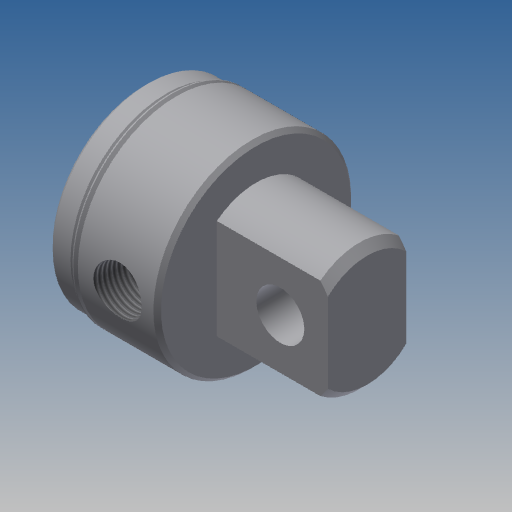
# Autodesk Inventor part: 17P0000_rear_head
Saved by Autodesk Inventor 2020 (Build 240168000, 168)
## iProperties
Created: 2020-02-18
Part Number: 17P0000_rear_head
Material: Generic
Catalog Web Link: www.cadenas.de
Description: Rear Head-Original Line - Standard Air Cylinders
Vendor: BIMBA
Document SubType Name: Modeling
Designer: psadmin
Manufacturer: BIMBA
Mass: 27.57 g
Surface Area: 88.2977 cm^2
Volume: 27.57 cm^3
Density: 1 g/cm^3
Appearance: PSOLRGB-211-211-211
Category: PARTsolutions
Company: BIMBA
PSOL_IDENT_0: {$CADENAS_DATA\23d-libs\bimba\bimba_brand\bimba_imperial\bimba_full_line\original_line_cylinders\sta
PSOL_IDENT_1: ndard_air_cylinders\rear_head.prj},239 {VTYP=3D},{NB=17P0000_rear_head},{LINA=17P0000_rear_head},{NN=
PSOL_IDENT_2: Rear Head},{DATE=10.02.2020 11:56:01},{GEOMDATE=15.10.2019 12:00:43},{VERSION=},{LINEID=80},{WBVAR=M
PSOL_IDENT_3: NT,ACTING,DER,Q,T1,T2,T3,T4,TRIM,Y,K,MB,CUSH,FBON},{WBNUMERIC=TRIM,MB,CUSH}  {NB=17P0000_rear_head},
PSOL_IDENT_4: {LINA=17P0000_rear_head},{KT=DUMMY},{PN=17P0000},{BORE=1.50000},{BOREPN=17},{MNT=P},{MNTALG='' , 'Fr
PSOL_IDENT_5: ont Nose' , 'P' , 'Rear Pivot' , 'S' , 'Built-in Valve S' , 'DX' , 'Double End' , 'A' , 'Adjustable
PSOL_IDENT_6: Stroke' , 'M' , 'Manual Valve' , 'BR' , 'Rear Block' , 'BRT' , 'Rear Trunnion'},{ACTING=},{ACTINGALG=
PSOL_IDENT_7: '' , 'Single Acting' },{DER=},{DERALG= '' , 'Standard' },{Q=},{T1=},{T2=},{T3=},{T4=},{TRIM=0},{Y=}
PSOL_IDENT_8: ,{K=},{KALG= '', 'without K', 'K', 'with K' },{MB=0},{A1=1.7500},{A1N=0.6880},{A1P=1.7500},{A1B=1.37
PSOL_IDENT_9: 50},{A1S=1.5000},{A2=0.25},{A2N=0.2500},{A3=0.0400},{D1=1.5565},{D1N=1.5565},{D1P=1.5565},{D1B=1.580
PSOL_IDENT_10: 0},{D2=1.5115},{C1=0.0300},{C2=0.0300},{NDM=0.4050},{TAB=NPT},{NDMDP=0.2730},{D3=0.3440},{A4=0.2500}
PSOL_IDENT_11: ,{A5=0.8700},{D4=0.9730},{A6=0.2500},{A7=0.6250},{A8=0.0000},{D5=0.0000},{D6=0.5320},{A9=0.7320},{ND
PSOL_IDENT_12: M2=0.0000},{TAB2=-},{C11=0.0300},{C22=0.0000},{C33=0.0000},{C44=0.0300},{A10=0.6170},{A11=0.0000},{N
PSOL_IDENT_13: DM3=0.4050},{NDM3N=0.4050},{NDM3B=0.5400},{TAB3=NPT},{TAB3N=NPT},{TAB3B=NPT},{A12=0.562},{A12N=0.562
PSOL_IDENT_14: 0},{A12B=0.7500},{A13=1.3750},{D7=0.3775},{D8=1.0000},{A14=0.0000},{A15=0.0000},{D9=0.0000},{R1=0.00
PSOL_IDENT_15: 00},{X1=0.9690},{X2=0.2500},{CX=0.0600},{CC=0.0000},{CON=1},{S1=1.7500},{DB=0.4380},{X1B=0.9730},{X2
PSOL_IDENT_16: B=0.2500},{A8B=0.1250},{A9B=1.0620},{MODEL=1},{NDM4=0.2500},{TAB4=UNC},{NDM4DP=0.5000},{BC=1.7500},{
PSOL_IDENT_17: B1=0.8750},{B2=0.3800},{B3=0.5000},{ON=0},{ON2=1},{G1=0.0000},{G2=0.0000},{G3=0.0000},{G4=0.0000},{G
PSOL_IDENT_18: D=0.0000},{G5=0.0000},{G6=0.0000},{RON=0},{H1=1.6160},{H2=1.5800},{H3=0.1250},{H4=0.1250},{H5=1.5300
PSOL_IDENT_19: },{H6=0.8120},{F=0.6240},{PNUT=0.0000},{CUSH=0},{CC11=0.397},{CC111=0.3965},{CC22=0.5625},{CC33=0.30
PSOL_IDENT_20: 50},{CC44=0.6250},{CC55=0.8750},{CD1=0.2650},{CD2=0.1980},{CD3=0.1345},{CNDM3=0.2500},{CTAB3=UNS},{O
PSOL_IDENT_21: LEN=1.3750},{OD=0.5025},{STDIS=0.3184},{STDIS1=0.3184},{BUSHCON=D-624},{BUSHL=0.7500},{FBON=0},{LCD=
PSOL_IDENT_22: 0.0000}
NN: Rear Head
NT: Original Line - Standard Air Cylinders
NB: 17P0000_rear_head
NBSYN: $PN._rear_head
LINA: 17P0000_rear_head
PN: 17P0000
BORE: 1.5
BOREPN: 17
MNT: Rear Pivot
MNTALG: '' , 'Front Nose' , 'P' , 'Rear Pivot' , 'S' , 'Built-in Valve S' , 'DX' , 'Double End' , 'A' , 'Adjustable Stroke' , 'M' , 'Manual Valve' , 'BR' , 'Rear Block' , 'BRT' , 'Rear Trunnion'
ACTING: Single Acting
DER: Standard
Q: Without Side Ported Rear Head
T1: without T1
T2: without T2
T3: without T3
T4: without T4
TRIM: 0
Y: without Pivot Bushing
K: without K
MB: 0
A1N: 0.688
A1P: 1.75
A1B: 1.375
A1S: 1.5
A2N: 0.25
A3: 0.04
D1N: 1.5565
D1P: 1.5565
D1B: 1.58
D2: 1.5115
C1: 0.03
C2: 0.03
TAB: NPT
NDMDP: 0.273
D3: 0.344
A4: 0.25
A5: 0.87
D4: 0.973
A6: 0.25
A7: 0.625
A8: 0
D5: 0
D6: 0.532
A9: 0.732
NDM2: 0
TAB2: -
C11: 0.03
C22: 0
C33: 0
C44: 0.03
A10: 0.617
A11: 0
NDM3N: 0.405
NDM3B: 0.54
TAB3N: NPT
TAB3B: NPT
A12N: 0.562
A12B: 0.75
A13: 1.375
D7: 0.3775
D8: 1
A14: 0
A15: 0
D9: 0
R1: 0
X1: 0.969
X2: 0.25
CX: 0.06
CC: 0
S1: 1.75
DB: 0.438
X1B: 0.973
X2B: 0.25
A8B: 0.125
A9B: 1.062
NDM4: 0.25
TAB4: UNC
NDM4DP: 0.5
BC: 1.75
B1: 0.875
B2: 0.38
B3: 0.5
G1: 0
G2: 0
G3: 0
G4: 0
GD: 0
G5: 0
G6: 0
H2: 1.58
H3: 0.125
F: 0.624
CUSH: 0
CC111: 0.3965
CC22: 0.5625
CC33: 0.305
CC44: 0.625
CC55: 0.875
CD1: 0.265
CD2: 0.198
CD3: 0.1345
CNDM3: 0.25
CTAB3: UNS
OD: 0.5025
STDIS1: 0.3184
BUSHCON: D-624
BUSHL: 0.75
FBON: 0
LCD: 0
SUPPLIER: BIMBA
ARTICLENO: 17P0000_rear_head
BOMINFO: 17P0000_rear_head
CREATOR: CADENAS GmbH
Title: 17P0000_rear_head
Author: Cadenas PARTsolutions
Comments: Original Line - Standard Air Cylinders
Autodesk Inventor part; units mm, degrees
sketch "Sketch_18" plane through (0, 0, 0) normal (0, 0, 1) x (1, 0, 0)
  line L0 (22.225, 0) -> (0, 0)
  line L1 (0, 0) -> (0, 18.434)
  line L2 (0, 18.434) -> (0.762, 19.196)
  line L3 (0.762, 19.196) -> (4.318, 19.196)
  line L4 (4.318, 19.196) -> (5.334, 18.1801)
  line L5 (5.334, 18.1801) -> (6.35, 18.1801)
  line L6 (6.35, 18.1801) -> (6.35, 19.7675)
  line L7 (6.35, 19.7675) -> (21.463, 19.7675)
  line L8 (21.463, 19.7675) -> (22.225, 19.0055)
  line L9 (22.225, 19.0055) -> (22.225, 0)
  line L10 (22.225, 0) -> (0, 0)
  constraints: 22 end point
revolve "Revolution1" add sketch "Sketch_18" angle 360 about axis through (22.225, 0, 0) along (1, 0, 0)
sketch "Sketch_21" plane through (0, 0, 0) normal (0, 0, 1) x (1, 0, 0)
  line L0 (44.45, 0) -> (22.225, 0)
  line L1 (22.225, 0) -> (22.225, 12.7)
  line L2 (22.225, 12.7) -> (42.926, 12.7)
  line L3 (42.926, 12.7) -> (44.45, 11.176)
  line L4 (44.45, 11.176) -> (44.45, 0)
  line L5 (44.45, 0) -> (22.225, 0)
  constraints: 12 end point
revolve "Revolution2" add sketch "Sketch_21" angle 360 about axis through (44.45, 0, 0) along (1, 0, 0)
sketch "Sketch_9" plane through (44.45, 0, 0) normal (1, 0, 0) x (0, 0, -1)
  line L0 (-39.5351, -79.0702) -> (39.5351, -79.0702)
  line L1 (39.5351, -79.0702) -> (39.5351, 79.0702)
  line L2 (39.5351, 79.0702) -> (-39.5351, 79.0702)
  line L3 (-39.5351, 79.0702) -> (-39.5351, -79.0702)
  line L4 (-7.8359, -39.5351) -> (7.8359, -39.5351)
  line L5 (7.8359, -39.5351) -> (7.8359, 39.5351)
  line L6 (7.8359, 39.5351) -> (-7.8359, 39.5351)
  line L7 (-7.8359, 39.5351) -> (-7.8359, -39.5351)
  constraints: 16 end point
extrude "Extrusion1" cut sketch "Sketch_9" against normal blind 22.225
sketch "Sketch4" plane through (0, 0, 0) normal (-1, 0, 0) x (0, 0, 1)
  point P0 (0, 0)
hole "Hole1" at (0, 0, 0) direction (1, 0, 0) diameter 13.5128 depth 20.4521 tip angle 120
sketch "Sketch_68" plane through (0, 0, 0) normal (0, 0.9998477, 0.0174524) x (1, 0, 0)
  line L0 (14.2748, -19.7675) -> (14.2748, 0)
  line L1 (14.2748, 0) -> (18.8978, 0)
  line L2 (18.8978, 0) -> (18.8978, -12.8333)
  line L3 (18.8978, -12.8333) -> (19.1143, -19.7675)
  line L4 (19.1143, -19.7675) -> (14.2748, -19.7675)
  line L5 (14.2748, -19.7675) -> (14.2748, 0)
  constraints: 12 end point
revolve "Revolution3" cut sketch "Sketch_68" angle 360 about axis through (14.2748, -0.345, 19.7645) along (0, -0.0174524, 0.9998477)
thread "Thread1" size "1/8" designation "1/8 - 27 NPT" standard "NPT" length 6.9376
sketch "Sketch_20" plane through (0, 0, 0) normal (0, 0, 1) x (1, 0, 0)
  line L0 (6.35, 0) -> (0, 0)
  line L1 (0, 0) -> (0, 12.3063)
  line L2 (0, 12.3063) -> (6.35, 12.3063)
  line L3 (6.35, 12.3063) -> (6.35, 0)
  line L4 (6.35, 0) -> (0, 0)
  constraints: 10 end point
revolve "Revolution4" cut sketch "Sketch_20" angle 360 about axis through (6.35, 0, 0) along (1, 0, 0)
sketch "Sketch_24" plane through (0, 0, 0) normal (0, 0, 1) x (1, 0, 0)
  line L0 (6.35, 0) -> (5.334, 0)
  line L1 (5.2675, 19.7675) -> (5.2675, 19.6834)
  line L2 (5.2675, 19.6834) -> (6.2166, 18.7343)
  arc A0 (6.2166, 18.5547) -> (6.2166, 18.7343) centre (6.1268, 18.6445) ccw
  line L3 (6.2166, 18.5547) -> (5.842, 18.1801)
  line L4 (5.842, 18.1801) -> (5.334, 18.1801)
  line L5 (5.334, 18.1801) -> (5.334, 17.9261)
  line L6 (5.334, 17.9261) -> (6.35, 17.9261)
  line L7 (6.35, 17.9261) -> (6.35, 18.8883)
  line L8 (6.35, 18.8883) -> (5.4707, 19.7675)
  line L9 (5.4707, 19.7675) -> (5.2675, 19.7675)
  constraints: 20 end point, 2 point on circle, 1 centre point
revolve "Revolution5" add sketch "Sketch_24" angle 360 about axis through (6.35, 0, 0) along (1, 0, 0)
sketch "Sketch_43" plane through (0, 0, 0) normal (0, 0, 1) x (1, 0, 0)
  circle A0 centre (34.925, 0) radius 4.7942
  constraints: 1 centre point
extrude "Extrusion2" cut sketch "Sketch_43" along normal mid plane 23.5077
ref_plane "f_XY" through (22.225, 0, 0) normal (0, 0, 1) x (1, 0, 0)
ref_plane "f_YZ" through (22.225, 0, 0) normal (1, 0, 0) x (0, 1, 0)
ref_plane "f_ZX" through (22.225, 0, 0) normal (0, 1, 0) x (0, 0, 1)
ref_plane "lovra1_XY" through (38.1, 0, 0) normal (1, 0, 0) x (0, 0, -1)
ref_plane "lovra1_YZ" through (38.1, 0, 0) normal (0, 0, -1) x (0, 1, 0)
ref_plane "lovra1_ZX" through (38.1, 0, 0) normal (0, 1, 0) x (1, 0, 0)
ref_plane "lovra2_XY" through (38.1, 11.049, 0) normal (1, 0, 0) x (0, 0, -1)
ref_plane "lovra2_YZ" through (38.1, 11.049, 0) normal (0, 0, -1) x (0, 1, 0)
ref_plane "lovra2_ZX" through (38.1, 11.049, 0) normal (0, 1, 0) x (1, 0, 0)
ref_plane "lovra21_XY" through (0, 0, 5.2705) normal (1, 0, 0) x (0, 0, -1)
ref_plane "lovra21_YZ" through (0, 0, 5.2705) normal (0, 0, -1) x (0, 1, 0)
ref_plane "lovra21_ZX" through (0, 0, 5.2705) normal (0, 1, 0) x (1, 0, 0)
ref_plane "lovra22_XY" through (0, 0, -5.2705) normal (1, 0, 0) x (0, 0, -1)
ref_plane "lovra22_YZ" through (0, 0, -5.2705) normal (0, 0, -1) x (0, 1, 0)
ref_plane "lovra22_ZX" through (0, 0, -5.2705) normal (0, 1, 0) x (1, 0, 0)
ref_plane "lovra3_XY" through (38.1, -11.049, 0) normal (1, 0, 0) x (0, 0, -1)
ref_plane "lovra3_YZ" through (38.1, -11.049, 0) normal (0, 0, -1) x (0, 1, 0)
ref_plane "lovra3_ZX" through (38.1, -11.049, 0) normal (0, 1, 0) x (1, 0, 0)
ref_plane "olen_XY" through (34.925, 0, 0) normal (1, 0, 0) x (0, 0, -1)
ref_plane "olen_YZ" through (34.925, 0, 0) normal (0, 0, -1) x (0, 1, 0)
ref_plane "olen_ZX" through (34.925, 0, 0) normal (0, 1, 0) x (1, 0, 0)
ref_plane "p1_XY" through (44.45, 0, 7.8359) normal (1, 0, 0) x (0, 0, -1)
ref_plane "p1_YZ" through (44.45, 0, 7.8359) normal (0, 0, -1) x (0, 1, 0)
ref_plane "p1_ZX" through (44.45, 0, 7.8359) normal (0, 1, 0) x (1, 0, 0)
ref_plane "p2_XY" through (44.45, 0, -7.8359) normal (1, 0, 0) x (0, 0, -1)
ref_plane "p2_YZ" through (44.45, 0, -7.8359) normal (0, 0, -1) x (0, 1, 0)
ref_plane "p2_ZX" through (44.45, 0, -7.8359) normal (0, 1, 0) x (1, 0, 0)
ref_plane "port_XY" through (14.2748, 0, 0) normal (0, 0, 1) x (1, 0, 0)
ref_plane "port_YZ" through (14.2748, 0, 0) normal (1, 0, 0) x (0, 1, 0)
ref_plane "port_ZX" through (14.2748, 0, 0) normal (0, 1, 0) x (0, 0, 1)
ref_plane "port2_XY" through (44.45, 0, 0) normal (1, 0, 0) x (0, 0, -1)
ref_plane "port2_YZ" through (44.45, 0, 0) normal (0, 0, -1) x (0, 1, 0)
ref_plane "port2_ZX" through (44.45, 0, 0) normal (0, 1, 0) x (1, 0, 0)
ref_plane "thd1_XY" through (44.45, 0, 0) normal (1, 0, 0) x (0, 0, -1)
ref_plane "thd1_YZ" through (44.45, 0, 0) normal (0, 0, -1) x (0, 1, 0)
ref_plane "thd1_ZX" through (44.45, 0, 0) normal (0, 1, 0) x (1, 0, 0)
ref_plane "thd2_XY" through (44.45, 0, 0) normal (1, 0, 0) x (0, 0, -1)
ref_plane "thd2_YZ" through (44.45, 0, 0) normal (0, 0, -1) x (0, 1, 0)
ref_plane "thd2_ZX" through (44.45, 0, 0) normal (0, 1, 0) x (1, 0, 0)
ref_plane "to_mounting_bracket_XY" through (22.225, 0, 0) normal (1, 0, 0) x (0, 0, -1)
ref_plane "to_mounting_bracket_YZ" through (22.225, 0, 0) normal (0, 0, -1) x (0, 1, 0)
ref_plane "to_mounting_bracket_ZX" through (22.225, 0, 0) normal (0, 1, 0) x (1, 0, 0)
ref_plane "to_nut_XY" through (0, 0, 0) normal (1, 0, 0) x (0, 0, -1)
ref_plane "to_nut_YZ" through (0, 0, 0) normal (0, 0, -1) x (0, 1, 0)
ref_plane "to_nut_ZX" through (0, 0, 0) normal (0, 1, 0) x (1, 0, 0)
ref_plane "to_pin_XY" through (34.925, 0, 0) normal (0, 0, 1) x (1, 0, 0)
ref_plane "to_pin_YZ" through (34.925, 0, 0) normal (1, 0, 0) x (0, 1, 0)
ref_plane "to_pin_ZX" through (34.925, 0, 0) normal (0, 1, 0) x (0, 0, 1)
ref_plane "to_screw_XY" through (14.2748, 14.2875, -10.0838) normal (0, 1, 0) x (1, 0, 0)
ref_plane "to_screw_YZ" through (14.2748, 14.2875, -10.0838) normal (1, 0, 0) x (0, 0, -1)
ref_plane "to_screw_ZX" through (14.2748, 14.2875, -10.0838) normal (0, 0, -1) x (0, 1, 0)
ref_plane "to_tube_XY" through (5.334, 0, 0) normal (1, 0, 0) x (0, 0, -1)
ref_plane "to_tube_YZ" through (5.334, 0, 0) normal (0, 0, -1) x (0, 1, 0)
ref_plane "to_tube_ZX" through (5.334, 0, 0) normal (0, 1, 0) x (1, 0, 0)
body "Solid1"
